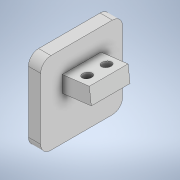
# Autodesk Inventor part: BrakeShoeWithTilt_Base
Saved by Autodesk Inventor 2022 (Build 260153000, 153)
## iProperties
Created: 2022-05-04
Part Number: BrakeShoeWithTilt_Base
Material: Generic
Document SubType Name: Modeling
Designer: NIC
Density: 1 g/cm^3
Appearance: Default
Author: NIC
Autodesk Inventor part; units mm, degrees
ref_plane "YZ Plane" through (0, 0, 0) normal (1, 0, 0) x (0, 1, 0)
ref_plane "XZ Plane" through (0, 0, 0) normal (0, 1, 0) x (-1, 0, 0)
sketch "Sketch1" plane through (0, 0, 0) normal (1, 0, 0) x (0, 1, 0)
  line L0 (-12.7, 12.7) -> (12.7, 12.7)
  line L1 (12.7, 12.7) -> (12.7, -12.7)
  line L2 (12.7, -12.7) -> (-12.7, -12.7)
  line L3 (-12.7, -12.7) -> (-12.7, 12.7)
  line L4 (-12.7, 12.7) -> (12.7, -12.7) construction
  line L5 (12.7, 12.7) -> (-12.7, -12.7) construction
  point P0 (0, 0)
  dimension "d0" = 25.4
  dimension "d1" = 25.4
  constraints: 12 end point, 2 midpoint, 2 parallel, 1 horizontal, 1 perpendicular
  measures "d0" distance of L1.end L2.end
  measures "d1" distance of L0.end L1.end
extrude "Extrusion1" add sketch "Sketch1" along normal blind 3.81
ref_plane "Work Plane2" through (3.81, 12.7, -12.7) normal (0.9925462, 0.1218693, 0) x (0, 0, 1)
sketch "Sketch2" plane through (5.3342, 0.2862, 0) normal (0.9925462, 0.1218693, 0) x (0, 0, -1)
  line L0 (-6, 0.7324) -> (6, 0.7324)
  line L1 (6, 0.7324) -> (6, 5.7324)
  line L2 (6, 5.7324) -> (-6, 5.7324)
  line L3 (-6, 5.7324) -> (-6, 0.7324)
  line L4 (-6, 0.7324) -> (6, 5.7324) construction
  line L5 (6, 0.7324) -> (-6, 5.7324) construction
  point P0 (0, 0.366)
  point P1 (0, 3.2324)
  dimension "d4" = 12
  dimension "d5" = 5
  constraints: 12 end point, 2 midpoint, 2 parallel, 1 horizontal, 1 perpendicular
  measures "d4" distance of L2.end L1.end
  measures "d5" distance of L1.end L0.end
extrude "Extrusion2" add sketch "Sketch2" along normal blind 7.62
sketch "Sketch3" plane through (3.81, 5.8744, 6) normal (-0.1218693, 0.9925462, 0) x (0.9925462, 0.1218693, 0)
  line L0 (8.4518, 12) -> (8.4518, 0) projected
  line L1 (13.7995, 6) -> (-14.4563, 6) projected
  point P0 (-4.4975, 6)
  point P1 (4.7518, 3)
  dimension "d8" = 3.7
  dimension "d9" = 3
  measures "d8" distance from line of L0 point (4.752, 3)
  measures "d9" distance from line of L1 point (4.752, 3)
hole "Hole1" at (8.5264, 6.4535, 3) direction (0.1218693, -0.9925462, 0) diameter 2.8956 end through all clearance for "Flat Head Machine Screw" size "M2.5" standard "Ansi Metric M Profile"
mirror "Mirror1" about plane through (0, 0, 0) normal (0, 0, 1) of "Hole1"
sketch "Sketch4" plane through (0, 0, 0) normal (0, 0, 1) x (1, 0, 0)
  arc A0 (2.54, 0) -> (-200.66, 0) centre (-99.06, 0) ccw
  line L0 (0, 12.7) -> (0, -12.7) projected
  line L1 (-241.3, 0) -> (43.18, 0) projected
  line L2 (-200.66, 0) -> (2.54, 0)
  line L3 (-241.3, 0) -> (43.18, 0) projected
  point P0 (0, 0)
  dimension "d17" = 203.2
  dimension "d18" = 99.06
  constraints: 2 end point, 2 point on circle, 2 point on line, 1 centre point, 1 midpoint
  measures "d17" diameter of A0
  measures "d18" distance from line of L0 A0.centre
revolve "Revolution1" [suppressed]
fillet "Fillet1" radius 3.175 4 edges at (1.905, 12.7, -12.7) (1.905, 12.7, 12.7) (1.905, -12.7, 12.7) (1.905, -12.7, -12.7)
fillet "Fillet2" [suppressed]
sketch "Sketch5" plane through (5.3342, 0.2862, 0) normal (-0.9925462, -0.1218693, 0) x (0, 0, 1)
  line L0 (-6, 0.7324) -> (-6, 5.7324) projected
  line L1 (6, 0.7324) -> (-6, 0.7324) projected
  line L2 (6, 5.7324) -> (6, 0.7324) projected
  line L3 (-6, 5.7324) -> (6, 5.7324) projected
  point P0 (0, 0.366)
extrude "Extrusion3" add sketch "Sketch5" along normal up to surface surface through (3.81, 0, 0) normal (1, 0, 0)
ref_plane "Work Plane1" through (0, 0, 0) normal (0, 0, 1) x (1, 0, 0)
body "Solid1"
